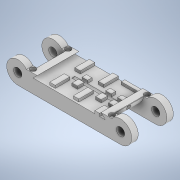
# Autodesk Inventor part: mPalm
Saved by Autodesk Inventor 2020 (Build 240168000, 168)
## iProperties
Created: 2019-10-21
Part Number: mPalm
Material: Generic
Document SubType Name: Modeling
Designer: ayad493
Density: 1 g/cm^3
Appearance: Default
Author: ayad493
Autodesk Inventor part; units mm, degrees
ref_plane "YZ Plane" through (0, 0, 0) normal (1, 0, 0) x (0, 1, 0)
ref_plane "XZ Plane" through (0, 0, 0) normal (0, 1, 0) x (-1, 0, 0)
ref_plane "XY Plane" through (0, 0, 0) normal (0, 0, 1) x (1, 0, 0)
sketch "Sketch1" plane through (0, 0, 0) normal (0, 0, 1) x (1, 0, 0)
  line L0 (0, 0) -> (-74, 0)
  line L1 (-74, 0) -> (-74, 5)
  line L2 (-74, 5) -> (0, 5)
  line L3 (0, 5) -> (0, 0)
  circle A0 centre (-74, 0) radius 8
  circle A1 centre (0, 0) radius 8
  line L4 (-74, 0) -> (0, 0)
  line L5 (0, 0) -> (0, 1)
  line L6 (0, 1) -> (-74, 1)
  line L7 (-74, 1) -> (-74, 0)
  point P0 (-74, 4)
  point P1 (-66.0627, 1)
  point P2 (-7.9373, 1)
  point P3 (0, 4)
  point P4 (-66, 0)
  point P5 (-67.755, 5)
  point P6 (-6.245, 5)
  point P7 (-8, 0)
  dimension "d0" = 74
  dimension "d1" = 5
  dimension "d2" = 16
  dimension "d3" = 16
  dimension "d4" = 1
  constraints: 16 end point, 4 parallel, 2 centre point, 2 coincident, 2 horizontal, 2 perpendicular, 1 point on line
  measures "d0" distance of L1.end L2.end
  measures "d1" distance of L0.end L1.end
  measures "d2" diameter of A0
  measures "d3" diameter of A1
  measures "d4" distance of L5.end L4.end
extrude "Extrusion1" add sketch "Sketch1" along normal blind 30 contours A0 L2 L1 L0 | L0 L1 L6 A0 | A1 L6 L3 L0 | L0 L3 L2 A1 | L6 L1 L2 A0 | A0 L2 A1 L6 | A1 L2 L3 L6
sketch "Sketch3" plane through (0, 0, 30) normal (0, 0, 1) x (1, 0, 0)
  circle A0 centre (0, 0) radius 3
  arc A1 (-67.755, 5) -> (-66.0627, 1) centre (-74, 0) ccw projected
  circle A2 centre (-74, 0) radius 3
  dimension "d8" = 6
  dimension "d9" = 6
  constraints: 2 centre point, 2 coincident
  measures "d8" diameter of A0
  measures "d9" diameter of A2
extrude "Extrusion2" cut sketch "Sketch3" against normal through all
sketch "Sketch6" plane through (-66.0627, 1, 0) normal (0, -1, 0) x (1, 0, 0)
  line L0 (-15.9373, 0) -> (-15.9373, 30) projected
  line L1 (-15.9373, 30) -> (0.0627, 30)
  line L2 (0.0627, 30) -> (0.0627, 25.3)
  line L3 (0.0627, 25.3) -> (-15.9373, 25.3)
  line L4 (-15.9373, 25.3) -> (-15.9373, 30)
  line L5 (58.0627, 30) -> (74.0627, 30)
  line L6 (58.0627, 25.3) -> (58.0627, 30)
  line L7 (74.0627, 25.3) -> (58.0627, 25.3)
  line L8 (74.0627, 30) -> (74.0627, 25.3)
  line L9 (-15.9373, 4.7) -> (0.0627, 4.7)
  line L10 (-15.9373, 0) -> (-15.9373, 4.7)
  line L11 (0.0627, 0) -> (-15.9373, 0)
  line L12 (0.0627, 4.7) -> (0.0627, 0)
  line L13 (58.0627, 4.7) -> (74.0627, 4.7)
  line L14 (58.0627, 0) -> (58.0627, 4.7)
  line L15 (74.0627, 0) -> (58.0627, 0)
  line L16 (74.0627, 4.7) -> (74.0627, 0)
  line L17 (-15.9373, 25.3) -> (0.0627, 25.3)
  line L18 (0.0627, 25.3) -> (0.0627, 4.7)
  line L19 (0.0627, 4.7) -> (-15.9373, 4.7)
  line L20 (-15.9373, 4.7) -> (-15.9373, 25.3)
  line L21 (74.0627, 25.3) -> (58.0627, 25.3)
  line L22 (58.0627, 25.3) -> (58.0627, 4.7)
  line L23 (58.0627, 4.7) -> (74.0627, 4.7)
  line L24 (74.0627, 4.7) -> (74.0627, 25.3)
  line L25 (0.0627, 25.3) -> (1.0627, 25.3)
  line L26 (1.0627, 25.3) -> (1.0627, 4.7)
  line L27 (1.0627, 4.7) -> (0.0627, 4.7)
  line L28 (0.0627, 4.7) -> (0.0627, 25.3)
  line L29 (58.0627, 25.3) -> (57.0627, 25.3)
  line L30 (57.0627, 25.3) -> (57.0627, 4.7)
  line L31 (57.0627, 4.7) -> (58.0627, 4.7)
  line L32 (58.0627, 4.7) -> (58.0627, 25.3)
  point P0 (66.0627, 0)
  point P1 (0.0627, 25.3)
  point P2 (0.0627, 4.7)
  dimension "d26" = 16
  dimension "d27" = 4.7
  dimension "d30" = 74
  dimension "d33" = 25.3
  dimension "d36" = 1
  dimension "d37" = 1
  constraints: 64 end point, 10 parallel, 6 horizontal, 5 perpendicular, 2 collinear, 2 point on line, 1 vertical, 22 other
  measures "d26" distance of L2.end L3.end
  measures "d27" distance of L1.end L2.end
  measures "d30" distance of L1.start L5.start
  measures "d33" distance of L1.start L9.start
  measures "d36" distance of L26.end L27.end
  measures "d37" distance of L31.end L30.end
extrude "Extrusion4" cut sketch "Sketch6" along normal blind 30 and the other way blind 15 contours L0 L3 L18 L9 | L18 L25 L26 L27 | L7 L24 L13 L22 | L22 L31 L30 L29
sketch "Sketch7" plane through (0, 0, 30) normal (0, 0, 1) x (1, 0, 0)
  circle A0 centre (0, 0) radius 3 projected
  arc A1 (-67.755, 5) -> (-66.0627, 1) centre (-74, 0) ccw projected
  line L0 (0, 0) -> (-74, 0)
  line L1 (-74, 0) -> (-74, -8)
  line L2 (-74, -8) -> (0, -8)
  line L3 (0, -8) -> (0, 0)
  circle A2 centre (-74, 0) radius 3 projected
  circle A3 centre (-74, 0) radius 8
  circle A4 centre (0, 0) radius 8
  point P0 (-8, 0)
  point P1 (-66, 0)
  constraints: 8 end point, 2 coincident, 2 parallel, 1 centre point, 1 horizontal, 1 perpendicular, 1 point on circle, 3 other
extrude "Extrusion5" add sketch "Sketch7" against normal blind 4.7 contours A4 L2 A1 L0
sketch "Sketch8" plane through (0, 0, 0) normal (0, 0, -1) x (-1, 0, 0)
  line L0 (0, -8) -> (74, -8) projected
  line L1 (0, 0) -> (74, 0)
  line L2 (74, 0) -> (74, -8)
  line L3 (74, -8) -> (0, -8)
  line L4 (0, -8) -> (0, 0)
  circle A0 centre (0, 0) radius 8
  circle A1 centre (74, 0) radius 8
  point P0 (66, 0)
  point P1 (8, 0)
  constraints: 8 end point, 2 centre point, 2 coincident, 2 parallel, 1 horizontal, 1 perpendicular
extrude "Extrusion6" add sketch "Sketch8" against normal blind 4.7 contours A0 L1 A1 L0
sketch "Sketch11" plane through (-66.0627, 1, 0) normal (0, -1, 0) x (1, 0, 0)
  line L0 (57.0627, 4.7) -> (57.0627, 25.3) projected
  line L1 (58.0627, 4.7) -> (0.0627, 4.7) projected
  line L2 (57.0627, 25.3) -> (1.0553, 25.3)
  line L3 (1.0553, 25.3) -> (1.0553, 4.7)
  line L4 (1.0553, 4.7) -> (57.0627, 4.7)
  line L5 (57.0627, 4.7) -> (57.0627, 25.3)
  point P0 (66.0627, 0)
  constraints: 8 end point, 2 parallel, 1 horizontal, 1 perpendicular, 1 point on line
extrude "Extrusion7" add sketch "Sketch11" along normal blind 2
sketch "Sketch12" plane through (0, 0, 0) normal (0, 0, -1) x (-1, 0, 0)
  arc A0 (8, 0) -> (7.9373, 1) centre (0, 0) ccw projected
  line L0 (7.9373, 1) -> (66.0627, 1)
  line L1 (66.0627, 1) -> (66.0627, 0)
  line L2 (66.0627, 0) -> (7.9373, 0)
  line L3 (7.9373, 0) -> (7.9373, 1)
  constraints: 8 end point, 2 parallel, 1 horizontal, 1 perpendicular
extrude "Extrusion8" add sketch "Sketch12" against normal blind 4.7
sketch "Sketch13" plane through (0, 0, 30) normal (0, 0, 1) x (1, 0, 0)
  line L0 (-7.9373, 1) -> (-66.0627, 1)
  line L1 (-66.0627, 1) -> (-66.0627, 0)
  line L2 (-66.0627, 0) -> (-7.9373, 0)
  line L3 (-7.9373, 0) -> (-7.9373, 1)
  point P0 (0, 0)
  constraints: 8 end point, 2 parallel, 1 horizontal, 1 perpendicular
extrude "Extrusion9" add sketch "Sketch13" against normal blind 4.7
fillet "Fillet1" radius 5.5 2 edges at (-9, -1, 15) (-65.0074, -1, 15)
sketch "Sketch14" plane through (0, 0, 30) normal (0, 0, 1) x (1, 0, 0)
  line L0 (-65, 5) -> (-60, 5)
  line L1 (-6.245, 5) -> (-67.755, 5) projected
  line L2 (-6.245, 5) -> (-9, 5) projected
  line L3 (-9, 5) -> (-14, 5)
  line L4 (-14, 5) -> (-14, 10)
  line L5 (-60, 10) -> (-60, 5)
  line L6 (-55, 10) -> (-60, 5)
  line L7 (-19, 10) -> (-14, 5)
  line L8 (-37, 10) -> (-37, 7)
  arc A0 (-55, 10) -> (-19, 10) centre (-37, 62.5) ccw
  line L9 (-60, 5) -> (-14, 5)
  line L10 (-14, 5) -> (-14, 2)
  line L11 (-14, 2) -> (-60, 2)
  line L12 (-60, 2) -> (-60, 5)
  line L13 (-60, 5) -> (-63, 2)
  line L14 (-63, 2) -> (-60, 2)
  line L15 (-14, 5) -> (-11, 2)
  line L16 (-11, 2) -> (-14, 2)
  line L17 (-60, 5) -> (-14, 5)
  line L18 (-36.7599, 5) -> (-41.7599, 5)
  point P0 (0, 0)
  dimension "d53" = 5
  dimension "d54" = 5
  dimension "d60" = 3
  dimension "d63" = 3
  dimension "d64" = 5
  constraints: 34 end point, 6 perpendicular, 6 point on line, 4 equal length, 3 point on circle, 2 horizontal, 1 centre point
  measures "d53" distance of L0.start L0.end
  measures "d54" distance of L2.end L3.end
  measures "d60" distance of L8.start L8.end
  measures "d63" distance of L9.end L10.end
  measures "d64" distance of L18.start L18.end
extrude "Extrusion12" cut sketch "Sketch14" against normal blind 30 contours L10 L11 L12 L1 | L15 L16 L10 | L14 L13 L12
sketch "Sketch15" plane through (-63, 2, 30) normal (0, 1, 0) x (1, 0, 0)
  line L0 (0, 30) -> (52, 30) projected
  line L1 (0, 30) -> (3, 30)
  line L2 (3, 30) -> (12.5, 30)
  line L3 (12.5, 30) -> (12.5, 21.5)
  line L4 (10.5, 19.5) -> (14.5, 19.5)
  line L5 (14.5, 19.5) -> (14.5, 23.5)
  line L6 (14.5, 23.5) -> (10.5, 23.5)
  line L7 (10.5, 23.5) -> (10.5, 19.5)
  line L8 (10.5, 19.5) -> (14.5, 23.5) construction
  line L9 (14.5, 19.5) -> (10.5, 23.5) construction
  line L10 (14.5, 19.5) -> (10.5, 19.5)
  line L11 (10.5, 19.5) -> (10.5, 30)
  line L12 (10.5, 30) -> (14.5, 30)
  line L13 (14.5, 30) -> (14.5, 19.5)
  line L14 (14.5, 19.5) -> (19, 19.5)
  line L15 (19, 19.5) -> (23, 19.5)
  line L16 (23, 19.5) -> (23, 9)
  line L17 (23, 9) -> (19, 9)
  line L18 (19, 9) -> (19, 19.5)
  line L19 (27.5, 30) -> (31.5, 30)
  line L20 (27.5, 19.5) -> (27.5, 30)
  line L21 (31.5, 30) -> (31.5, 19.5)
  line L22 (27.5, 19.5) -> (31.5, 19.5)
  line L23 (10.5, 12) -> (14.5, 12)
  line L24 (10.5, 1.5) -> (10.5, 12)
  line L25 (14.5, 12) -> (14.5, 1.5)
  line L26 (10.5, 1.5) -> (14.5, 1.5)
  line L27 (27.5, 12) -> (31.5, 12)
  line L28 (27.5, 1.5) -> (27.5, 12)
  line L29 (31.5, 12) -> (31.5, 1.5)
  line L30 (27.5, 1.5) -> (31.5, 1.5)
  line L31 (52, 0) -> (0, 0) projected
  line L32 (10.5, 0) -> (14.5, 0)
  line L33 (27.5, 0) -> (31.5, 0)
  line L34 (36, 19.5) -> (40, 19.5)
  line L35 (36, 9) -> (36, 19.5)
  line L36 (40, 19.5) -> (40, 9)
  line L37 (40, 9) -> (36, 9)
  line L38 (40, 19.5) -> (44.5, 19.5)
  line L39 (44.5, 19.5) -> (47.9548, 19.5)
  line L40 (47.9548, 19.5) -> (47.9548, 0)
  line L41 (47.9548, 0) -> (44.5, 0)
  line L42 (44.5, 0) -> (44.5, 19.5)
  line L43 (44.5, 9.75) -> (47.9548, 9.75)
  line L44 (47.9548, 9.75) -> (47.9548, 6.75)
  line L45 (47.9548, 6.75) -> (44.5, 6.75)
  line L46 (44.5, 6.75) -> (44.5, 9.75)
  point P0 (63, 30)
  point P1 (44.5, 6.75)
  point P2 (27.5, 1.5)
  point P3 (10.5, 1.5)
  point P4 (10.5, 30)
  point P5 (10.5, 23.5)
  point P6 (14.5, 23.5)
  point P7 (14.5, 30)
  dimension "d67" = 3
  dimension "d68" = 9.5
  dimension "d69" = 8.5
  dimension "d70" = 4
  dimension "d71" = 4
  dimension "d72" = 4.5
  dimension "d73" = 4
  dimension "d74" = 10.5
  dimension "d77" = 17
  dimension "d80" = 18
  dimension "d85" = 17
  dimension "d90" = 4.5
  constraints: 90 end point, 13 point on line, 10 parallel, 9 horizontal, 6 perpendicular, 3 collinear, 3 midpoint, 1 vertical, 32 other
  measures "d67" distance of L0.start L1.end
  measures "d68" distance of L1.end L2.end
  measures "d69" distance of L2.end L3.end
  measures "d70" distance of L6.end L5.end
  measures "d71" distance of L5.end L4.end
  measures "d72" distance of L4.end L14.end
  measures "d73" distance of L16.end L17.end
  measures "d74" distance of L15.end L16.end
  measures "d77" distance of L11.end L19.start
  measures "d80" distance of L11.end L23.start
  measures "d85" distance of L14.end L34.start
  measures "d90" distance of L34.end L38.end
extrude "Extrusion13" add sketch "Sketch15" along normal blind 1.9 contours L0 L3 L6 L11 | L0 L13 L6 L3 | L6 L5 L4 L7 | L0 L21 L22 L20 | L15 L16 L17 L18 | L23 L25 L26 L24 | L27 L29 L30 L28 | L31 L42 L45 L40 | L43 L42 L39 L40 | L34 L36 L37 L35
sketch "Sketch16" plane through (-9, 5, 25.3) normal (1, 0, 0) x (0, 0, -1)
  line L0 (20.6, 0) -> (0, 0) projected
  line L1 (10.3, 0) -> (10.3, -6)
  line L2 (20.6, -6) -> (0, -6) projected
  line L3 (0, -4) -> (20.6, -4) projected
  line L4 (10.3, -4) -> (10.3, 0)
  circle A0 centre (10.3, -2) radius 1.5
  point P0 (25.3, -5)
  constraints: 4 end point, 4 midpoint, 1 centre point, 1 vertical
extrude "Extrusion14" cut sketch "Sketch16" against normal blind 40
sketch "Sketch17" plane through (-67.755, 5, 4.7) normal (0, 1, 0) x (1, 0, 0)
  line L0 (0, -20.6) -> (0, -25.3) projected
  line L1 (67.755, -20.6) -> (-6.245, -20.6) projected
  line L2 (0, -25.3) -> (4.7, -25.3)
  line L3 (4.7, -25.3) -> (4.7, -20.6)
  line L4 (4.7, -20.6) -> (0, -20.6)
  line L5 (0, -20.6) -> (0, -25.3)
  line L6 (0, 4.7) -> (0, 0) projected
  line L7 (67.755, 4.7) -> (-6.245, 4.7) projected
  line L8 (0, 0) -> (4.7, 0)
  line L9 (4.7, 0) -> (4.7, 4.7)
  line L10 (4.7, 4.7) -> (0, 4.7)
  line L11 (0, 4.7) -> (0, 0)
  line L12 (61.51, 4.7) -> (61.51, 0) projected
  line L13 (61.51, 0) -> (56.81, 0)
  line L14 (56.81, 0) -> (56.81, 4.7)
  line L15 (56.81, 4.7) -> (61.51, 4.7)
  line L16 (61.51, 4.7) -> (61.51, 0)
  line L17 (61.51, -20.6) -> (61.51, -25.3) projected
  line L18 (-6.245, -25.3) -> (67.755, -25.3) projected
  line L19 (61.51, -20.6) -> (56.81, -20.6)
  line L20 (56.81, -20.6) -> (56.81, -25.3)
  line L21 (56.81, -25.3) -> (61.51, -25.3)
  line L22 (61.51, -25.3) -> (61.51, -20.6)
  line L23 (7.755, -25.3) -> (0, -25.3) projected
  line L24 (4.7, -20.6) -> (0, -25.3)
  line L25 (4.7, 0) -> (0, 4.7)
  line L26 (56.81, 0) -> (61.51, 4.7)
  line L27 (56.81, -20.6) -> (61.51, -25.3)
  circle A0 centre (59.16, -22.95) radius 2
  circle A1 centre (59.16, 2.35) radius 2
  circle A2 centre (2.35, 2.35) radius 2
  circle A3 centre (2.35, -22.95) radius 2
  dimension "d96" = 4.7
  dimension "d97" = 4.7
  dimension "d98" = 4.7
  dimension "d99" = 4.7
  dimension "d102" = 4
  dimension "d103" = 4
  dimension "d104" = 4
  dimension "d105" = 4
  constraints: 40 end point, 8 parallel, 5 perpendicular, 5 point on line, 4 centre point, 4 horizontal, 4 midpoint
  measures "d96" distance of L4.end L3.end
  measures "d97" distance of L10.end L9.end
  measures "d98" distance of L14.end L15.end
  measures "d99" distance of L21.end L20.end
  measures "d102" diameter of A0
  measures "d103" diameter of A1
  measures "d104" diameter of A2
  measures "d105" diameter of A3
extrude "Extrusion16" cut sketch "Sketch17" against normal blind 2 contours A3 L24 | L24 A3 | A0 L27 | L27 A0 | A2 L25 | L25 A2 | A1 L26 | L26 A1
sketch "Sketch18" plane through (-63, 2, 30) normal (0, 1, 0) x (1, 0, 0)
  line L0 (36, 16.118) -> (36, 19.5) projected
  line L1 (36, 19.5) -> (36, 30)
  line L2 (63, 30) -> (-11, 30) projected
  line L3 (36, 30) -> (48, 30)
  line L4 (48, 30) -> (48, 27.5)
  line L5 (48, 27.5) -> (36, 27.5)
  line L6 (36, 27.5) -> (36, 30)
  dimension "d108" = 12
  dimension "d109" = 2.5
  constraints: 10 end point, 2 parallel, 1 horizontal, 1 perpendicular, 1 point on line, 1 vertical
  measures "d108" distance of L4.end L5.end
  measures "d109" distance of L3.end L4.end
extrude "Extrusion17" add sketch "Sketch18" along normal blind 1.9
body "Solid1"
